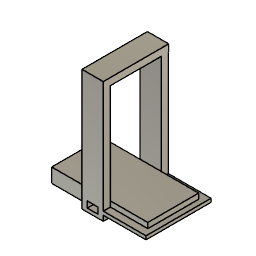
Camera+Mount (2) (Autodesk Fusion 360 design; units mm, degrees)
part number: 2025-10-27-17-01-54-419
Autodesk Fusion 360 part; units mm, degrees
sketch "Sketch2" plane through (0, 0, 0) normal (0, 0, 1) x (1, 0, 0)
  line L0 (0, 0) -> (685.8, 0)
  line L1 (685.8, 0) -> (685.8, 363.22)
  line L2 (685.8, 363.22) -> (0, 363.22)
  line L3 (0, 363.22) -> (0, 0)
  dimension "d1" = 685.8
  dimension "d2" = 363.22
  constraint horizontal L0
  constraint vertical L1
  constraint horizontal L2
  constraint vertical L3
  constraint coincident L0.start L3.end
  measures "d1" distance of L0.start L0.end
  measures "d2" distance of L0.start L2.end
extrude "Extrude1" add sketch "Sketch2" along normal blind 101.6
sketch "Sketch3" plane through (0, 0, 0) normal (0, 1, 0) x (1, 0, 0)
  line L0 (266.7, 0) -> (419.1, 0)
  line L1 (419.1, 0) -> (419.1, -812.8)
  line L2 (419.1, -812.8) -> (266.7, -812.8)
  line L3 (266.7, -812.8) -> (266.7, 0)
  dimension "d6" = 152.4
  dimension "d7" = 152.4
  dimension "d8" = 812.8
  constraint vertical L1
  constraint horizontal L2
  constraint vertical L3
  measures "d6" distance of L0.start L0.end
  measures "d7" distance of L0.start L0.end
  measures "d8" distance of L0.start L2.end
extrude "Extrude2" add sketch "Sketch3" against normal blind 50.8
sketch "Sketch8" plane through (0, 363.22, 0) normal (0, 1, 0) x (-1, 0, 0)
  line L0 (-685.8, 0) -> (0, 0)
  line L1 (0, 0) -> (0, 101.6)
  line L2 (0, 101.6) -> (-685.8, 101.6)
  line L3 (-685.8, 101.6) -> (-685.8, 0)
  line L4 (-419.1, 101.6) -> (-419.1, 0)
  line L5 (-266.7, 101.6) -> (-266.7, 0)
  line L6 (-419.1, 0) -> (-266.7, 0)
  line L7 (-266.7, 0) -> (-266.7, 812.8)
  line L8 (-266.7, 812.8) -> (-419.1, 812.8)
  line L9 (-419.1, 812.8) -> (-419.1, 0)
  dimension "d19" = 101.6
  dimension "d20" = 152.4
  dimension "d21" = 812.8
  constraint coincident L2 L4.start
  constraint coincident L0 L4.end
  constraint perpendicular L0 L4
  constraint coincident L2 L5.start
  constraint perpendicular L2 L5
  constraint horizontal L6
  constraint vertical L7
  constraint horizontal L8
  constraint vertical L9
  measures "d19" distance of L5.start L5.end
  measures "d20" distance of L4.end L5.end
  measures "d21" distance of L4.end L8.end
extrude "Extrude6" add sketch "Sketch8" along normal blind 50.8 contours L0 L2 L4 L5 L6 L7 L9 | L2 L7 L8 L9
sketch "Sketch9" plane through (0, 0, 812.8) normal (0, 0, 1) x (-1, 0, 0)
  line L0 (-419.1, 0) -> (-266.7, 0)
  line L1 (-266.7, 0) -> (-266.7, 50.8)
  line L2 (-266.7, 50.8) -> (-419.1, 50.8)
  line L3 (-419.1, 50.8) -> (-419.1, 0)
  line L4 (-419.1, 50.8) -> (-266.7, 50.8)
  line L5 (-266.7, 50.8) -> (-266.7, -416.56)
  line L6 (-266.7, -416.56) -> (-419.1, -416.56)
  line L7 (-419.1, -416.56) -> (-419.1, 50.8)
  constraint horizontal L4
  constraint vertical L5
  constraint horizontal L6
  constraint vertical L7
  constraint coincident L2.end L3.start
extrude "Extrude7" add sketch "Sketch9" along normal blind 50.8
sketch "Sketch11" plane through (0, -50.8, 0) normal (0, -1, 0) x (1, 0, 0)
  line L0 (266.7, 863.6) -> (266.7, 0)
  line L1 (419.1, 0) -> (419.1, 863.6)
  line L2 (419.1, 863.6) -> (266.7, 863.6)
  line L3 (0, 50.8) -> (304.8, 50.8)
  line L4 (685.8, 50.8) -> (381, 50.8)
  line L5 (381, 50.8) -> (304.8, 50.8)
  line L6 (342.9, 0) -> (342.9, 25.4)
  line L7 (342.9, 101.6) -> (342.9, 69.85)
  line L8 (304.8, 50.8) -> (381, 50.8)
  line L9 (381, 50.8) -> (381, 25.4)
  line L10 (381, 25.4) -> (304.8, 25.4)
  line L11 (304.8, 25.4) -> (304.8, 50.8)
  line L12 (304.8, 50.8) -> (381, 50.8)
  line L13 (381, 50.8) -> (381, 69.85)
  line L14 (381, 69.85) -> (304.8, 69.85)
  line L15 (304.8, 69.85) -> (304.8, 50.8)
  line L16 (266.7, 0) -> (419.1, 0)
  dimension "d29" = 304.8
  dimension "d30" = 304.8
  dimension "d31" = 25.4
  dimension "d33" = 31.75
  constraint perpendicular L0 L3
  constraint horizontal L4
  constraint parallel L3 L5
  constraint perpendicular L5 L6
  constraint parallel L0 L7
  constraint horizontal L8
  constraint vertical L9
  constraint horizontal L10
  constraint vertical L11
  constraint horizontal L12
  constraint vertical L13
  constraint horizontal L14
  constraint vertical L15
  measures "d29" distance of L3.start L3.end
  measures "d30" distance of L4.start L4.end
  measures "d31" distance of L6.start L6.end
  measures "d33" distance of L7.start L7.end
extrude "Extrude9" cut sketch "Sketch11" against normal blind 660.4 contours L5 L8 L12 L13 L14 L15 | L5 L8 L9 L10 L11 L12
sketch "Sketch12" plane through (419.1, 0, 0) normal (1, 0, 0) x (0, 1, 0)
  line L0 (363.22, 812.8) -> (363.22, 101.6)
  line L1 (363.22, 101.6) -> (363.22, 0)
  line L2 (363.22, 0) -> (414.02, 0)
  line L3 (414.02, 0) -> (414.02, 812.8)
  line L4 (416.56, 812.8) -> (416.56, 863.6)
  line L5 (416.56, 863.6) -> (-50.8, 863.6)
  line L6 (-50.8, 863.6) -> (-50.8, 0)
  line L7 (-50.8, 0) -> (0, 0)
  line L8 (0, 0) -> (0, 101.6)
  line L9 (0, 101.6) -> (0, 812.8)
  line L10 (414.02, 812.8) -> (416.56, 812.8)
  line L11 (0, 101.6) -> (0, 63.5)
  line L12 (0, 0) -> (0, 38.1)
  line L13 (0, 63.5) -> (-50.8, 63.5)
  line L14 (-50.8, 63.5) -> (-50.8, 38.1)
  line L15 (-50.8, 38.1) -> (0, 38.1)
  line L16 (0, 38.1) -> (0, 63.5)
  line L17 (0, 812.8) -> (363.22, 812.8)
  constraint coincident L8.end L9.start
  constraint coincident L8 L11.end
  constraint coincident L7.end L8.start
  constraint coincident L8 L12.end
  constraint horizontal L13
  constraint vertical L14
  constraint horizontal L15
  constraint vertical L16
  constraint coincident L6 L14.end
extrude "Extrude10" add sketch "Sketch12" along normal blind 304.8 contours L6 L8 L13 L14 L15 L16
extrude "Extrude11" add 1 faces at (698.5, 0, 46.5667) along direction (0, 1, 0) blind 414.02
extrude "Extrude14" add 1 faces at (685.8, 380.1533, 46.5667) along direction (-1, 0, 0) blind 266.7
